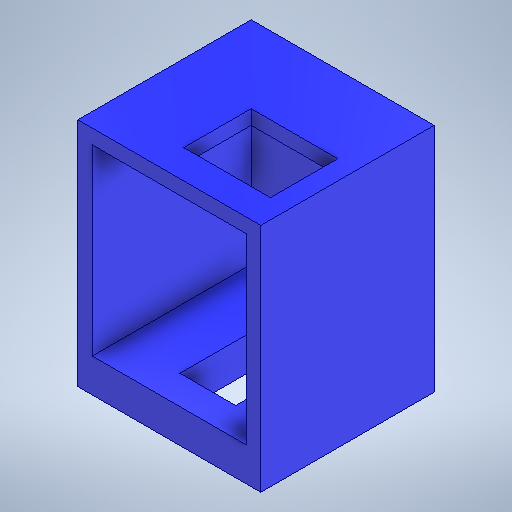
# Autodesk Inventor part: senzor_obal
Saved by Autodesk Inventor 2025.2 (Build 292293000, 293)
## iProperties
Created: 2025-03-02
Part Number: senzor_obal
Material: Všeobecné
Document SubType Name: Modeling
Designer: jakub
Density: 1 g/cm^3
Appearance: Modrá – nástěnná malba – lesklá
Author: jakub
## iProperties of the stored document senzor_obal_3D tisk.ipt
Created: 2025-03-02
Part Number: senzor_obal_3D tisk
Material: Všeobecné
Document SubType Name: Modeling
Designer: jakub
Density: 1 g/cm^3
Appearance: Výchozí
Author: jakub
Autodesk Inventor part; units mm, degrees
ref_plane "YZ Plane" through (0, 0, 0) normal (1, 0, 0) x (0, 1, 0)
ref_plane "XZ Plane" through (0, 0, 0) normal (0, 1, 0) x (-1, 0, 0)
ref_plane "XY Plane" through (0, 0, 0) normal (0, 0, 1) x (1, 0, 0)
sketch "Náčrt1" plane through (0, 0, 0) normal (0, 0, 1) x (1, 0, 0)
  line L0 (0, 18.2) -> (0, -18.2) projected
  line L1 (-14.7, 0) -> (14.7, 0) projected
  line L2 (-10.5, 13) -> (10.5, 13)
  line L3 (10.5, 13) -> (10.5, -13)
  line L4 (10.5, -13) -> (-10.5, -13)
  line L5 (-10.5, -13) -> (-10.5, 13)
  line L6 (-10.5, 13) -> (10.5, -13) construction
  line L7 (10.5, 13) -> (-10.5, -13) construction
  point P0 (0, 0)
  dimension "d0" = 21
  dimension "d1" = 26
  constraints: 12 end point, 2 midpoint, 2 parallel, 1 horizontal, 1 perpendicular
  measures "d0" distance of L3.end L4.end
  measures "d1" distance of L2.end L3.end
extrude "Vysunutí1" add sketch "Náčrt1" along normal blind 18
sketch "Náčrt4" plane through (0, 0, 18) normal (0, 0, 1) x (1, 0, 0)
  line L0 (-14.7, 0) -> (14.7, 0) projected
  line L1 (0, 18.2) -> (0, -18.2) projected
  line L2 (-10.5, -13) -> (10.5, -13) projected
  line L3 (10.5, -13) -> (10.5, 13) projected
  line L4 (10.5, 13) -> (-10.5, 13) projected
  line L5 (-10.5, 13) -> (-10.5, -13) projected
  line L6 (-9, -9.5) -> (7, -9.5)
  line L7 (7, -9.5) -> (7, 9.5)
  line L8 (7, 9.5) -> (-9, 9.5)
  line L9 (-9, 9.5) -> (-9, -9.5)
  point P0 (0, 0)
  dimension "d9" = 3.5
  dimension "d34" = 16
  dimension "d35" = 1.5
  dimension "d36" = 19
  constraints: 8 end point, 2 parallel, 1 horizontal, 1 perpendicular
  measures "d9" distance between parallel lines of L2 L6
  measures "d34" distance between parallel lines of L9 L7
  measures "d35" distance between parallel lines of L5 L9
  measures "d36" distance between parallel lines of L6 L8
extrude "Vysunutí2" cut sketch "Náčrt4" against normal blind 16.5 contours L9 L8 L1 L0 | L0 L1 L6 L9 | L1 L8 L7 L0 | L0 L7 L6 L1
sketch "Náčrt5" plane through (-10.5, 13, 0) normal (0, 1, 0) x (1, 0, 0)
  line L0 (21, 0) -> (0, 0) projected
  line L1 (0, 0) -> (0, -18) projected
  line L2 (21, -18) -> (0, -18) projected
  line L3 (21, 0) -> (21, -18) projected
  line L4 (17, -15) -> (8, -15)
  line L5 (8, -15) -> (8, -8)
  line L6 (8, -8) -> (17, -8)
  line L7 (17, -8) -> (17, -15)
  line L8 (17, -15) -> (8, -8) construction
  line L9 (8, -15) -> (17, -8) construction
  point P0 (10.5, 0)
  point P1 (12.5, -11.5)
  dimension "d12" = 9
  dimension "d13" = 7
  dimension "d14" = 3
  dimension "d15" = 8
  constraints: 12 end point, 2 midpoint, 2 parallel, 1 horizontal, 1 perpendicular
  measures "d12" distance of L5.end L6.end
  measures "d13" distance of L4.end L5.end
  measures "d14" distance between parallel lines of L2 L4
  measures "d15" distance between parallel lines of L1 L5
extrude "Vysunutí3" cut sketch "Náčrt5" against normal up to surface (3.5 mm away) contours L4 L5 L6 L7
sketch "Náčrt6" plane through (-10.5, -13, 0) normal (0, -1, 0) x (1, 0, 0)
  line L0 (0, 0) -> (21, 0) projected
  line L1 (21, 0) -> (21, 18) projected
  line L2 (0, 18) -> (21, 18) projected
  line L3 (0, 0) -> (0, 18) projected
  line L4 (7.6, 15) -> (13.4, 15)
  line L5 (13.4, 15) -> (13.4, 3)
  line L6 (13.4, 3) -> (7.6, 3)
  line L7 (7.6, 3) -> (7.6, 15)
  line L8 (7.6, 15) -> (13.4, 3) construction
  line L9 (13.4, 15) -> (7.6, 3) construction
  point P0 (10.5, 0)
  point P1 (10.5, 9)
  dimension "d18" = 5.8
  dimension "d19" = 12
  dimension "d20" = 10.5
  dimension "d21" = 9
  constraints: 12 end point, 2 midpoint, 2 parallel, 1 horizontal, 1 perpendicular
  measures "d18" distance of L5.end L6.end
  measures "d19" distance of L4.end L5.end
  measures "d20" distance from line of L1 point (10.5, 9)
  measures "d21" distance from line of L2 point (10.5, 9)
extrude "Vysunutí4" cut sketch "Náčrt6" against normal up to surface (3.5 mm away) contours L4 L5 L6 L7
sketch "Náčrt8" plane through (0, 0, 18) normal (0, 0, 1) x (1, 0, 0)
  line L0 (7, 9.5) -> (7, -9.5) projected
  line L1 (7, -9.5) -> (-9, -9.5) projected
  line L2 (-9, -9.5) -> (-9, 9.5) projected
  line L3 (-9, 9.5) -> (7, 9.5) projected
  line L4 (-10.5, -13) -> (10.5, -13) projected
  line L5 (10.5, -13) -> (10.5, 13) projected
  line L6 (10.5, 13) -> (-10.5, 13) projected
  line L7 (-10.5, 13) -> (-10.5, -13) projected
  line L8 (-10.5, 11) -> (8.5, 11)
  line L9 (8.5, -13) -> (8.5, 11)
  point P0 (0, 0)
  dimension "d37" = 1.5
  dimension "d38" = 1.5
  constraints: 4 end point, 2 point on line, 1 parallel, 1 perpendicular
  measures "d37" distance between parallel lines of L3 L8
  measures "d38" distance between parallel lines of L0 L9
extrude "Vysunutí6" cut sketch "Náčrt8" against normal through all contours L9 L8 L7 L6 L5 L4
